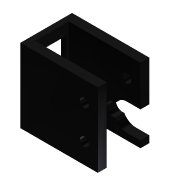
# Autodesk Inventor part: Greifer1
Saved by Autodesk Inventor 2015 (Build 190159000, 159)
## iProperties
Created: 2015-02-07
Part Number: Greifer1
Material: ABS-Kunststoff
Document SubType Name: Modeling
Designer: Luki
Density: 1.06 g/cm^3
Appearance: Glänzend - schwarz
Author: Luki
Autodesk Inventor part; units mm, degrees
ref_plane "YZ Plane" through (0, 0, 0) normal (1, 0, 0) x (0, 1, 0)
ref_plane "XZ Plane" through (0, 0, 0) normal (0, 1, 0) x (-1, 0, 0)
ref_plane "XY Plane" through (0, 0, 0) normal (0, 0, 1) x (1, 0, 0)
sketch "Skizze1" plane through (0, 0, 0) normal (1, 0, 0) x (0, 1, 0)
  line L0 (-6.5, 23) -> (-6.5, 0)
  line L1 (-6.5, 0) -> (6.5, 0)
  line L2 (6.5, 0) -> (6.5, 23)
  line L3 (6.5, 23) -> (-6.5, 23)
  line L4 (-6.5, 23) -> (6.5, 0) construction
  line L5 (-6.5, 0) -> (6.5, 23) construction
  line L6 (0, 34.6) -> (0, -11.6) projected
  line L7 (-16.1, 0) -> (16.1, 0) projected
  line L8 (-11.5, -5) -> (-11.5, 28)
  line L9 (-11.5, 28) -> (11.5, 28)
  line L10 (11.5, 28) -> (11.5, -5)
  line L11 (11.5, -5) -> (-11.5, -5)
  line L12 (-11.5, -5) -> (11.5, 28) construction
  line L13 (-11.5, 28) -> (11.5, -5) construction
  point P0 (0, 0)
  point P1 (0, 11.5)
  point P2 (0, 0)
  point P3 (0, 11.5)
  dimension "d0" = 23
  dimension "d1" = 13
  dimension "d2" = 5
  dimension "d3" = 5
  constraints: 24 end point, 8 midpoint, 4 parallel, 2 perpendicular, 1 vertical
  measures "d0" distance between parallel lines of L1 L3
  measures "d1" distance between parallel lines of L0 L2
  measures "d2" distance between parallel lines of L3 L9
  measures "d3" distance between parallel lines of L0 L8
extrude "Extrusion1" add sketch "Skizze1" along normal blind 2.5 contours L0 L7 L8 L9 L6 L3 | L1 L6 L11 L8 L7 | L6 L9 L10 L7 L2 L3 | L1 L7 L10 L11 L6
sketch "Skizze2" plane through (2.5, 0, 0) normal (1, 0, 0) x (0, 0, -1)
  line L0 (-23, 6.5) -> (-23, -6.5) projected
  line L1 (-23, -6.5) -> (0, -6.5) projected
  line L2 (0, -6.5) -> (0, 6.5) projected
  line L3 (0, 6.5) -> (-23, 6.5) projected
  line L4 (-28, -11.5) -> (-28, 11.5) projected
  line L5 (-28, 11.5) -> (5, 11.5) projected
  line L6 (5, 11.5) -> (5, -11.5) projected
  line L7 (5, -11.5) -> (-28, -11.5) projected
  line L8 (0, -16.1) -> (0, 16.1) projected
  line L9 (11.6, 0) -> (-34.6, 0) projected
  line L10 (-28, -11.5) -> (-28, 11.5) projected
  line L11 (5, -11.5) -> (-28, -11.5)
  line L12 (-28, -11.5) -> (-28, -7.5)
  line L13 (-28, -7.5) -> (5, -7.5)
  line L14 (5, -7.5) -> (5, -11.5)
  line L15 (5, 11.5) -> (-28, 11.5)
  line L16 (-28, 11.5) -> (-28, 7.5)
  line L17 (-28, 7.5) -> (5, 7.5)
  line L18 (5, 7.5) -> (5, 11.5)
  point P0 (0, 0)
  dimension "d6" = 4
  dimension "d7" = 4
  constraints: 16 end point, 4 parallel, 2 horizontal, 2 perpendicular, 2 point on line
  measures "d6" distance between parallel lines of L7 L13
  measures "d7" distance between parallel lines of L5 L17
extrude "Extrusion2" add sketch "Skizze2" along normal blind 32 contours L17 L4 L5 L8 | L8 L5 L6 L17 | L13 L8 L7 L4 | L13 L6 L7 L8
sketch "Skizze3" plane through (0, -11.5, -5) normal (0, -1, 0) x (1, 0, 0)
  line L0 (34.5, 33) -> (34.5, 0) projected
  line L1 (34.5, 0) -> (0, 0) projected
  line L2 (0, 0) -> (0, 33) projected
  line L3 (0, 33) -> (34.5, 33) projected
  line L4 (0, 39.6) -> (0, -6.6) projected
  circle A0 centre (28.5, 9) radius 7.5
  circle A1 centre (28.5, 24) radius 7.5
  circle A2 centre (28.5, 9) radius 2
  circle A3 centre (28.5, 24) radius 2
  point P0 (0, 5)
  dimension "d10" = 15
  dimension "d11" = 15
  dimension "d12" = 33
  dimension "d13" = 9
  dimension "d14" = 4
  dimension "d15" = 4
  dimension "d16" = 6
  dimension "d17" = 6
  constraints: 4 centre point, 2 coincident, 1 equal radius
  measures "d10" diameter of A0
  measures "d11" diameter of A1
  measures "d12" distance between parallel lines of L3 L1
  measures "d13" distance from line of L1 A0.centre
  measures "d14" diameter of A2
  measures "d15" diameter of A3
  measures "d16" distance from line of L0 A0.centre
  measures "d17" distance from line of L0 A1.centre
extrude "Extrusion3" cut sketch "Skizze3" against normal blind 40 contours A2 | A3
sketch "Skizze4" plane through (0, 11.5, 28) normal (0, 1, 0) x (1, 0, 0)
  circle A0 centre (28.5, 9) radius 2 projected
  circle A1 centre (28.5, 24) radius 2 projected
  line L0 (34.5, 33) -> (34.5, 0) projected
  line L1 (34.5, 0) -> (0, 0) projected
  line L2 (0, 0) -> (0, 33) projected
  line L3 (0, 33) -> (34.5, 33) projected
  circle A2 centre (28.5, 24) radius 2 projected
  circle A3 centre (28.5, 24) radius 6
  circle A4 centre (22.5, 24) radius 3
  line L4 (34.5, 33) -> (34.5, 0) projected
  line L5 (28.5, 18) -> (34.5, 18)
  line L6 (34.5, 18) -> (34.5, 30)
  line L7 (34.5, 30) -> (28.5, 30)
  line L8 (28.5, 30) -> (28.5, 18)
  point P0 (0, 28)
  dimension "d20" = 12
  dimension "d21" = 6
  dimension "d22" = 6
  constraints: 8 end point, 3 horizontal, 2 parallel, 1 centre point, 1 coincident, 1 perpendicular, 1 point on line, 1 vertical alignment, 2 other
  measures "d21" diameter of A4
  measures "d22" distance of A1.centre A4.centre
extrude "Extrusion4" cut sketch "Skizze4" against normal blind 5 contours A1 L8 | A1 L8 A3 | L8 A1 | A1 L8 A3 A4 | L7 L0 A3 | A3 L0 L5 | A4 A3 | A3 A4
sketch "Skizze5" plane through (0, 11.5, 28) normal (0, 1, 0) x (1, 0, 0)
  line L0 (0, 33) -> (11.5, 33)
  line L1 (11.5, 33) -> (11.5, 18)
  line L2 (11.5, 18) -> (0, 18)
  line L3 (0, 18) -> (0, 33)
  point P0 (0, 28)
  dimension "d25" = 11.5
  dimension "d26" = 15
  constraints: 8 end point, 2 parallel, 1 horizontal, 1 perpendicular
  measures "d25" distance between parallel lines of L3 L1
  measures "d26" distance between parallel lines of L0 L2
extrude "Extrusion5" add sketch "Skizze5" along normal blind 4.5
sketch "Skizze6" plane through (0, 16, 28) normal (0, 1, 0) x (1, 0, 0)
  line L0 (11.5, 33) -> (11.5, 18) projected
  line L1 (11.5, 18) -> (0, 18) projected
  line L2 (0, 18) -> (0, 33) projected
  line L3 (0, 33) -> (11.5, 33) projected
  circle A0 centre (8.8, 24) radius 1
  point P0 (0, 28)
  dimension "d29" = 2.7
  dimension "d30" = 9
  dimension "d31" = 2
  constraints: 1 centre point
  measures "d29" distance from line of L0 A0.centre
  measures "d30" distance from line of L3 A0.centre
  measures "d31" diameter of A0
extrude "Extrusion6" cut sketch "Skizze6" against normal blind 4.5 contours A0
equation "\"d13\" = 0 * d10 + 0.5 * d12 - 0.5 * d11"
equation "\"d17\" = d16"
